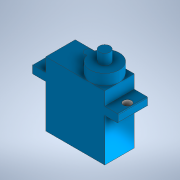
# Autodesk Inventor part: servo1
Saved by Autodesk Inventor 2021 (Build 250183000, 183)
## iProperties
Created: 2023-05-12
Part Number: servo1
Material: PBT Plastic
Document SubType Name: Modeling
Designer: shrus
Density: 1.31 g/cm^3
Appearance: Smooth - White
Mass: 6.99092 g
Surface Area: 25.7247 cm^2
Volume: 6.5458 cm^3
Sheet Metal Rule: Default
Author: shrus
Autodesk Inventor part; units mm, degrees
ref_plane "YZ Plane" through (0, 0, 0) normal (1, 0, 0) x (0, 1, 0)
ref_plane "XZ Plane" through (0, 0, 0) normal (0, 1, 0) x (-1, 0, 0)
ref_plane "XY Plane" through (0, 0, 0) normal (0, 0, 1) x (1, 0, 0)
sketch "Sketch1" plane through (0, 0, 0) normal (0, 0, 1) x (1, 0, 0)
  line L0 (-11.3443, 2.4351) -> (-0.3443, 2.4351)
  line L1 (-0.3443, 2.4351) -> (-0.3443, 26.4351)
  line L2 (-0.3443, 26.4351) -> (-11.3443, 26.4351)
  line L3 (-11.3443, 26.4351) -> (-11.3443, 2.4351)
  line L4 (-10.0022, 21.4351) -> (-10.0022, 22.9768)
  line L5 (-11.3443, 21.4351) -> (-16.0443, 21.4351)
  line L6 (-16.3443, 21.1351) -> (-16.3443, 18.7351)
  line L7 (-16.0443, 18.4351) -> (-11.3443, 18.4351)
  line L8 (10.6557, 2.4351) -> (-0.3443, 2.4351)
  line L9 (-0.3443, 26.4351) -> (10.6557, 26.4351)
  line L10 (10.6557, 26.4351) -> (10.6557, 2.4351)
  line L11 (10.6557, 21.4351) -> (15.3557, 21.4351)
  line L12 (15.6557, 21.1351) -> (15.6557, 18.7351)
  line L13 (15.3557, 18.4351) -> (10.6557, 18.4351)
  arc A0 (-16.3443, 18.7351) -> (-16.0443, 18.4351) centre (-16.0443, 18.7351) ccw
  arc A1 (-16.0443, 21.4351) -> (-16.3443, 21.1351) centre (-16.0443, 21.1351) ccw
  arc A2 (15.3557, 18.4351) -> (15.6557, 18.7351) centre (15.3557, 18.7351) ccw
  arc A3 (15.6557, 21.1351) -> (15.3557, 21.4351) centre (15.3557, 21.1351) ccw
  point P0 (0, 0)
  point P1 (-16.3443, 21.4351)
  point P2 (-16.3443, 18.4351)
  point P3 (15.6557, 21.4351)
  point P4 (15.6557, 18.4351)
  dimension "d0" = 11
  dimension "d1" = 24
  dimension "d3" = 5
  dimension "d4" = 3
  dimension "d5" = 0.3
  constraints: 28 end point, 12 point on line, 8 point on circle, 8 tangent, 6 symmetric about line, 4 centre point, 3 equal radius, 3 perpendicular, 2 vertical, 1 horizontal
  measures "d0" distance of L0.start L0.end
  measures "d1" distance of L0.end L1.end
  measures "d3" distance of L5.start point (-16.344, 21.435)
  measures "d4" distance of point (-16.344, 21.435) point (-16.344, 18.435)
  measures "d5" radius of A0
extrude "Extrusion1" add sketch "Sketch1" along normal mid plane 11
sketch "Sketch2" plane through (-11.3443, 26.4351, 5.5) normal (0, 1, 0) x (1, 0, 0)
  line L0 (22, 11) -> (22, 0) projected
  arc A0 (11.1667, 4.1563) -> (11.1667, 6.8437) centre (16.5, 5.5) ccw
  arc A1 (11.1667, 6.8437) -> (11.1667, 4.1563) centre (10.5, 5.5) ccw
  point P0 (11.3443, 5.5)
  dimension "d9" = 11
  dimension "d11" = 3
  constraints: 4 point on circle, 2 centre point
  measures "d9" diameter of A0
  measures "d11" diameter of A1
extrude "Extrusion2" add sketch "Sketch2" along normal blind 4
sketch "Sketch3" plane through (-11.3443, 30.4351, 5.5) normal (0, 1, 0) x (1, 0, 0)
  line L0 (22, 11) -> (22, 5.5) projected
  circle A0 centre (16.5, 5.5) radius 2
  point P0 (11.3443, 5.5)
  constraints: 1 centre point
extrude "Extrusion3" add sketch "Sketch3" along normal blind 4
sketch "Sketch4" plane through (-16.0443, 21.4351, 5.5) normal (0, 1, 0) x (1, 0, 0)
  point P0 (16.0443, 5.5)
  point P1 (1.5246, 5.3219)
  point P2 (29.8245, 5.3219)
hole "Hole1" at (13.7802, 21.4351, 0.1781) at (-14.5197, 21.4351, 0.1781) direction (0, -1, 0) diameter 3 end through all
equation "\"BendRadius\" = Thickness"
equation "\"BendReliefWidth\" = Thickness"
equation "\"BendReliefDepth\" = 0.5 * Thickness"
equation "\"CornerReliefSize\" = 4 * Thickness"
equation "\"MinimumRemnant\" = 2 * Thickness"
equation "\"TransitionRadius\" = BendRadius"
equation "\"JacobiRadiusSize\" = Thickness"
equation "\"GapSize\" = Thickness"
equation "\"Thickness\" = 0.5"
body "Solid1"
